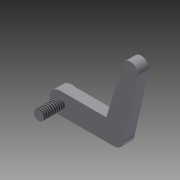
# Autodesk Inventor part: servo_hook
Saved by Autodesk Inventor 2015 SP2 (Build 190223200, 223)
## iProperties
Created: 2016-09-05
Part Number: servo_hook
Material: Generic
Document SubType Name: Modeling
Designer: jm799
Density: 1 g/cm^3
Appearance: Default
Author: jm799
Autodesk Inventor part; units mm, degrees
ref_plane "YZ Plane" through (0, 0, 0) normal (1, 0, 0) x (0, 1, 0)
ref_plane "XZ Plane" through (0, 0, 0) normal (0, 1, 0) x (-1, 0, 0)
ref_plane "XY Plane" through (0, 0, 0) normal (0, 0, 1) x (1, 0, 0)
sketch "Sketch1" plane through (0, 0, 0) normal (0, 1, 0) x (-1, 0, 0)
  circle A0 centre (0, 0) radius 2
  circle A1 centre (0, 0) radius 0.95
  circle A2 centre (-10.0688, 0.0006) radius 1.9997
  line L0 (-0.0618, -1.999) -> (-10.0688, -1.999)
  line L1 (-0.0618, 1.999) -> (-10.0686, 2.0003)
  circle A3 centre (-13.2373, 11.8352) radius 1.5
  line L2 (-8.0691, 0.0006) -> (-11.8022, 12.2717)
  line L3 (-12.0685, 0.0006) -> (-14.7373, 11.8352)
  dimension "d0" = 4
  dimension "d1" = 1.9
  dimension "d2" = 3
  constraints: 8 end point, 8 point on circle, 4 centre point, 3 tangent, 2 coincident
  measures "d0" diameter of A0
  measures "d1" diameter of A1
  measures "d2" diameter of A3
extrude "Extrusion1" add sketch "Sketch1" along normal blind 2 contours A0 | A0 L0 A2 L2 L1 | L2 A2 L1 | L1 A2 L3 A3 L2 | A2 L2 | A2 L2 | A3 L3 picked at (-13.7105, 11.7661)
sketch "Sketch2" plane through (0, 2, 0) normal (0, 1, 0) x (1, 0, 0)
  circle A0 centre (0, 0) radius 0.95
  constraints: 1 centre point, 1 coincident
extrude "Extrusion2" add sketch "Sketch2" against normal blind 6 and the other way blind 0.5
thread "Thread1" size "M2x0.4" class "6g" standard "ANSI Metric M Profile" full length
sketch "Sketch3" plane through (0, 2, 0) normal (0, 1, 0) x (1, 0, 0)
  circle A0 centre (0, 0) radius 1.8246
  constraints: 1 centre point, 1 coincident
extrude "Extrusion3" add sketch "Sketch3" along normal blind 0.3
body "Solid1"
